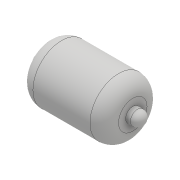
# Autodesk Inventor part: roller
Saved by Autodesk Inventor 2017 (Build 210142000, 142)
## iProperties
Created: 2018-10-27
Part Number: roller
Material: Generic
Document SubType Name: Modeling
Designer: mfans
Density: 1 g/cm^3
Appearance: Default
Author: mfans
Autodesk Inventor part; units mm, degrees
ref_plane "YZ Plane" through (0, 0, 0) normal (1, 0, 0) x (0, 1, 0)
ref_plane "XZ Plane" through (0, 0, 0) normal (0, 1, 0) x (-1, 0, 0)
ref_plane "XY Plane" through (0, 0, 0) normal (0, 0, 1) x (1, 0, 0)
sketch "Sketch1" plane through (0, 0, 0) normal (0, 0, 1) x (1, 0, 0)
  line L0 (-9, -6) -> (9, -6)
  line L1 (9, -6) -> (9, 6)
  line L2 (9, 6) -> (-9, 6)
  line L3 (-9, 6) -> (-9, 0)
  line L4 (-9, -6) -> (9, 6) construction
  line L5 (9, -6) -> (-9, 6) construction
  line L6 (-9, 0) -> (9, 0)
  point P0 (0, 0)
  dimension "d0" = 18
  dimension "d1" = 12
  constraints: 14 end point, 3 midpoint, 2 parallel, 1 horizontal, 1 perpendicular
  measures "d0" distance between parallel lines of L1 L3
  measures "d1" distance of L0.end L1.end
revolve "Revolution1" add sketch "Sketch1" angle 360 about axis through (-9, 0, 0) along (1, 0, 0)
sketch "Sketch2" plane through (9, 0, 0) normal (1, 0, 0) x (0, 0, -1)
  circle A0 centre (0, 0) radius 1.5
  dimension "d3" = 3
  constraints: 1 centre point, 1 coincident
  measures "d3" diameter of A0
extrude "Extrusion1" add sketch "Sketch2" along normal blind 2.5
fillet "Fillet1" radius 1.5 1 edges at (11.5, 0, 1.5)
mirror "Mirror1" about plane through (0, 0, 0) normal (1, 0, 0) of "Extrusion1"
fillet "Fillet2" radius 1.5 1 edges at (-11.5, 0, 1.5)
fillet "Fillet3" radius 3 2 edges at (-9, -6, 0) (9, -6, 0)
body "Solid1"
